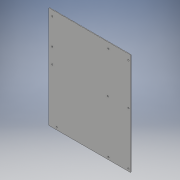
# Autodesk Inventor part: atxboard
Saved by Autodesk Inventor 2018 (Build 220112000, 112)
## iProperties
Created: 2021-04-25
Part Number: atxboard
Material: Generic
Document SubType Name: Modeling
Designer: gisen
Density: 1 g/cm^3
Appearance: Default
Author: gisen
Autodesk Inventor part; units mm, degrees
ref_plane "YZ Plane" through (0, 0, 0) normal (1, 0, 0) x (0, 1, 0)
ref_plane "XZ Plane" through (0, 0, 0) normal (0, 1, 0) x (-1, 0, 0)
ref_plane "XY Plane" through (0, 0, 0) normal (0, 0, 1) x (1, 0, 0)
sketch "Sketch1" plane through (0, 0, 0) normal (0, 1, 0) x (-1, 0, 0)
  line L0 (0, 0) -> (-244, 0)
  line L1 (-244, 0) -> (-244, -305)
  line L2 (-244, -305) -> (0, -305)
  line L3 (0, -305) -> (0, 0)
  dimension "d0" = 244
  dimension "d1" = 305
  constraints: 8 end point, 2 parallel, 1 horizontal, 1 perpendicular
  measures "d0" distance of L1.end L2.end
  measures "d1" distance of L0.end L1.end
extrude "Extrusion1" add sketch "Sketch1" along normal blind 1.651
sketch "Sketch2" plane through (0, 1.651, 0) normal (0, 1, 0) x (1, 0, 0)
  line L0 (0, 305) -> (0, 0) projected
  line L1 (0, 0) -> (244, 0) projected
  line L2 (244, 0) -> (244, 305) projected
  point P0 (10, 17)
  point P1 (10, 96)
  point P2 (10, 142)
  point P3 (238, 17)
  point P4 (177.9993, 17)
  point P5 (176.1481, 141)
  point P6 (178, 298)
  point P7 (23, 298)
  point P8 (238, 141)
  point P9 (238, 298)
  dimension "d4" = 10
  dimension "d5" = 17
  dimension "d6" = 79
  dimension "d8" = 46
  dimension "d11" = 6
  dimension "d14" = 17
  dimension "d16" = 155
  dimension "d17" = 23
  dimension "d18" = 124
  dimension "d19" = 157
  measures "d4" distance from line of L0 point (10, 17)
  measures "d5" distance from line of point (10, 17) L1
  measures "d6" distance of point (10, 17) point (10, 96)
  measures "d8" distance of point (10, 142) point (10, 96)
  measures "d11" distance from line of L2 point (238, 17)
  measures "d14" distance from line of point (177.999, 17) L1
  measures "d16" distance of point (178, 298) point (23, 298)
  measures "d17" distance from line of L0 point (23, 298)
  measures "d18" vertical distance of point (176.148, 141) point (177.999, 17)
  measures "d19" vertical distance of point (178, 298) point (176.148, 141)
hole "Hole1" at (10, 1.651, -17) at (10, 1.651, -96) at (10, 1.651, -142) at (238, 1.651, -17) at (177.9993, 1.651, -17) at (176.1481, 1.651, -141) at (178, 1.651, -298) at (23, 1.651, -298) at (238, 1.651, -141) at (238, 1.651, -298) direction (0, -1, 0) diameter 4 end through all
body "Solid1"
